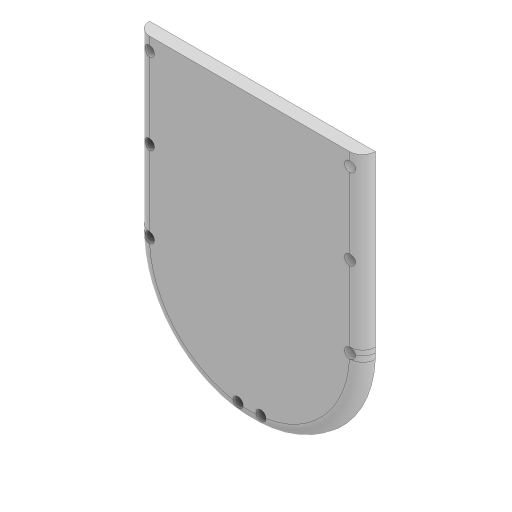
# Autodesk Inventor part: top plate front
Saved by Autodesk Inventor 2024 (Build 280153000, 153)
## iProperties
Created: 2024-08-03
Part Number: top plate front
Material: Generic
Document SubType Name: Modeling
Designer: chris
Density: 1 g/cm^3
Appearance: Default
Author: chris
Autodesk Inventor part; units mm, degrees
ref_plane "YZ Plane" through (0, 0, 0) normal (1, 0, 0) x (0, 1, 0)
ref_plane "XZ Plane" through (0, 0, 0) normal (0, 1, 0) x (-1, 0, 0)
ref_plane "XY Plane" through (0, 0, 0) normal (0, 0, 1) x (1, 0, 0)
sketch "Sketch1" plane through (0, 0, 0) normal (0, 0, 1) x (1, 0, 0)
  arc A0 (44.4535, 146.5784) -> (40.443, 154.3447) centre (34.9285, 146.5784) ccw
  arc A1 (40.443, 154.3447) -> (-40.436, 154.3447) centre (0.0035, 97.3915) ccw
  arc A2 (-40.436, 154.3447) -> (-44.4465, 146.5784) centre (-34.9215, 146.5784) ccw
  line L0 (-44.4465, 146.5784) -> (-44.4465, 24.273)
  arc A3 (-44.4465, 24.273) -> (44.4535, 24.273) centre (0.0035, 24.273) ccw
  line L1 (44.4535, 24.273) -> (44.4535, 146.5784)
  circle A4 centre (-4.5, -14.5) radius 2
  circle A5 centre (-39.3665, 24.273) radius 2
  circle A6 centre (39.3735, 24.273) radius 2
  circle A7 centre (4.5, -14.5) radius 2
  circle A8 centre (-39.3665, 56.023) radius 2
  circle A9 centre (-39.3665, 87.773) radius 2
  circle A10 centre (-39.3665, 132.223) radius 2
  circle A11 centre (0.0035, 162.1615) radius 2
  circle A12 centre (39.3735, 56.023) radius 2
  circle A13 centre (39.3735, 87.773) radius 2
  circle A14 centre (39.3735, 132.223) radius 2
  line L2 (-39.3665, 87.773) -> (-39.3665, 92.853)
  line L3 (-44.4465, 92.853) -> (44.4535, 92.853)
  point P0 (0, 0)
  point P1 (0, 0)
  dimension "d5" = 5.08
  constraints: 15 centre point, 8 end point, 8 point on circle, 2 point on line, 1 horizontal, 1 parallel
  measures "d5" distance of L2.start L2.end
extrude "Extrusion1" add sketch "Sketch1" along normal blind 5.08 contours L1 A3 L0 L3
fillet "Fillet1" radius 5.08 3 edges at (-44.4465, 58.563, 5.08) (0.0035, -20.177, 5.08) (44.4535, 58.563, 5.08)
body "Solid1"
